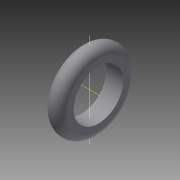
# Autodesk Inventor part: Part3
Saved by Autodesk Inventor 2015 (Build 190159000, 159)
## iProperties
Created: 2015-01-14
Part Number: Part3
Material: Generic
Document SubType Name: Modeling
Designer: admin
Density: 1 g/cm^3
Appearance: Default
Author: admin
Autodesk Inventor part; units mm, degrees
ref_plane "YZ Plane" through (0, 0, 0) normal (1, 0, 0) x (0, 1, 0)
ref_plane "XZ Plane" through (0, 0, 0) normal (0, 1, 0) x (-1, 0, 0)
ref_plane "XY Plane" through (0, 0, 0) normal (0, 0, 1) x (1, 0, 0)
sketch "Sketch1" plane through (0, 0, 0) normal (0, 1, 0) x (-1, 0, 0)
  line L0 (12, -35) -> (-12, -35)
  line L1 (-12, -35) -> (-12, -55)
  line L2 (-12, -55) -> (12, -55)
  line L3 (12, -55) -> (12, -35)
  line L4 (0, -66) -> (0, 11) construction
  line L5 (16.8, 0) -> (-16.8, 0) construction
  point P0 (0, 0)
  point P1 (0, -35)
  dimension "d1" = 24
  dimension "d2" = 35
  dimension "d3" = 55
  constraints: 8 end point, 2 parallel, 1 horizontal, 1 midpoint, 1 perpendicular, 1 other
  measures "d1" distance of L1.end L2.end
  measures "d2" distance between parallel lines of L5 L0
  measures "d3" distance from line of point (0, 0) L2
revolve "Revolution1" add sketch "Sketch1" angle 360 about axis through (-10, 0, 0) along (1, 0, 0)
fillet "Fillet1" radius 12 2 edges at (12, 0, 55) (-12, 0, 55)
body "Solid1"
